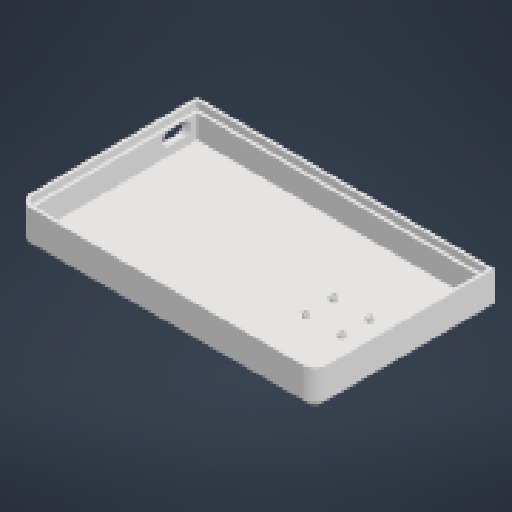
# Autodesk Inventor part: AASTRC Bottom case
Saved by Autodesk Inventor 2024 (Build 280153000, 153)
## iProperties
Created: 2023-07-16
Part Number: AASTRC Bottom case
Material: 일반
Document SubType Name: Modeling
Designer: 6gioc
Density: 1 g/cm^3
Appearance: 기본값
Mass: 597.29 g
Surface Area: 2047.87 cm^2
Volume: 597.29 cm^3
Author: 6gioc
Autodesk Inventor part; units mm, degrees
ref_plane "YZ Plane" through (0, 0, 0) normal (1, 0, 0) x (0, 1, 0)
ref_plane "XZ Plane" through (0, 0, 0) normal (0, 1, 0) x (-1, 0, 0)
ref_plane "XY Plane" through (0, 0, 0) normal (0, 0, 1) x (1, 0, 0)
sketch "스케치1" plane through (0, 0, 0) normal (0, 1, 0) x (-1, 0, 0)
  line L0 (0, 0) -> (217, 0)
  line L1 (217, 0) -> (217, -131)
  line L2 (217, -131) -> (0, -131)
  line L3 (0, -131) -> (0, 0)
  dimension "d0" = 217
  dimension "d1" = 131
  constraints: 8 end point, 2 parallel, 1 horizontal, 1 perpendicular
  measures "d0" distance of L1.end L2.end
  measures "d1" distance of L0.end L1.end
extrude "돌출1" add sketch "스케치1" along normal blind 27
sketch "스케치8" plane through (0, 27, -131) normal (0, 0, -1) x (-1, 0, 0)
  line L0 (0, -27) -> (217, -27) projected
  line L1 (217, -27) -> (217, 0) projected
  line L2 (0, 0) -> (217, 0) projected
  line L3 (0, -27) -> (0, 0) projected
  point P0 (0, -27)
extrude "돌출7" add sketch "스케치8" along normal blind 50
sketch "스케치9" plane through (0, 27, 0) normal (0, 1, 0) x (1, 0, 0)
  line L0 (0, 181) -> (-217, 181) projected
  line L1 (0, 0) -> (0, 181) projected
  line L2 (-217, 181) -> (0, 181)
  line L3 (0, 181) -> (0, 154)
  line L4 (0, 154) -> (-217, 154)
  line L5 (-217, 154) -> (-217, 181)
  point P0 (0, 10)
  dimension "d56" = 27
  constraints: 8 end point, 2 parallel, 1 horizontal, 1 perpendicular, 1 point on line
  measures "d56" distance of L2.end L3.end
extrude "돌출8" add sketch "스케치9" along normal blind 154
fillet "모깎기5" radius 10 4 edges at (-217, 181, -167.5) (0, 181, -167.5) (-217, 13.5, 0) (0, 13.5, 0)
chamfer "모따기3" distance 23 angle 45 1 edges at (-108.5, 27, -154)
shell "쉘3" thickness 10 removed faces 3 at (-141.3333, 93.6667, -154) at (-144.6667, 42.3333, -146.3333) at (-141.3333, 27, -87.3333)
sketch "스케치12" plane through (-207, 10, -171) normal (0, 0, 1) x (1, 0, 0)
  line L0 (0, 0) -> (0, 161) projected
  line L1 (197, 0) -> (0, 0) projected
  line L2 (197, 0) -> (197, 161) projected
  line L3 (197, 161) -> (0, 161) projected
  point P0 (207, -10)
extrude "돌출11" cut sketch "스케치12" against normal blind 5
sketch "스케치13" plane through (-207, 10, -10) normal (0, 1, 0) x (1, 0, 0)
  line L0 (0, 0) -> (197, 0) projected
  line L1 (197, 0) -> (197, 166) projected
  line L2 (197, 166) -> (0, 166) projected
  line L3 (0, 0) -> (0, 166) projected
  point P0 (207, -10)
extrude "돌출12" cut sketch "스케치13" against normal blind 5
chamfer "모따기4" distance 10 angle 45 1 edges at (-108.5, 5, -176)
sketch "스케치15" plane through (-207, 10, -176) normal (0, 0, 1) x (1, 0, 0)
  line L0 (73.5, 105.5) -> (123.5, 105.5)
  line L1 (123.5, 105.5) -> (123.5, 55.5)
  line L2 (123.5, 55.5) -> (73.5, 55.5)
  line L3 (73.5, 55.5) -> (73.5, 105.5)
  line L4 (197, 5) -> (0, 5) projected
  line L5 (197, 161) -> (197, 5) projected
  line L6 (0, 161) -> (197, 161) projected
  line L7 (0, 5) -> (0, 161) projected
  line L8 (197, 161) -> (197, 40) projected
  line L9 (197, 161) -> (197, 5) projected
  arc A0 (207, 161) -> (197, 171) centre (197, 161) ccw projected
  line L10 (207, -10) -> (207, 161) projected
  line L11 (207, -10) -> (-10, -10) projected
  line L12 (-10, -10) -> (-10, 161) projected
  arc A1 (0, 171) -> (-10, 161) centre (0, 161) ccw projected
  line L13 (197, 171) -> (0, 171) projected
  point P0 (98.5, 105.5)
  point P1 (73.5, 80.5)
  dimension "d85" = 50
  dimension "d86" = 50
  dimension "d87" = 197
  dimension "d88" = 156
  dimension "d89" = 98.5
  dimension "d90" = 181
  dimension "d91" = 90.5
  constraints: 8 end point, 2 midpoint, 2 parallel, 1 horizontal, 1 perpendicular
  measures "d85" distance of L1.end L2.end
  measures "d86" distance of L0.end L1.end
  measures "d87" distance of L6.start L5.start
  measures "d88" distance of L4.end L6.start
  measures "d89" distance from line of point (98.5, 105.5) L7
  measures "d90" distance between parallel lines of L11 L13
  measures "d91" distance from line of L13 point (73.5, 80.5)
extrude "돌출13" cut sketch "스케치15" against normal blind 4 contours L0 L1 L2 L3
sketch "스케치17" plane through (0, 27, -181) normal (0, 0, -1) x (-1, 0, 0)
  line L0 (133.5, 88.5) -> (133.5, 38.5) construction
  line L1 (133.5, 38.5) -> (83.5, 38.5) construction
  line L2 (83.5, 38.5) -> (83.5, 88.5) construction
  line L3 (83.5, 88.5) -> (133.5, 88.5) construction
  arc A0 (10, 154) -> (0, 144) centre (10, 144) ccw projected
  line L4 (0, -27) -> (0, 144) projected
  line L5 (0, -27) -> (217, -27) projected
  line L6 (217, -27) -> (217, 144) projected
  arc A1 (217, 144) -> (207, 154) centre (207, 144) ccw projected
  line L7 (10, 154) -> (207, 154) projected
  spline S0 degree 2 poles (123.7612, 75.7515) (121.8873, 75.1553) (119.3603, 70.6408) (119.3603, 68.4829) knots 0 0 0 1 2 2 2
  spline S1 degree 2 poles (119.3603, 68.4829) (119.3603, 65.7572) (122.2564, 61.0156) (124.5846, 60.3909) knots 0 0 0 1 2 2 2
  spline S2 degree 2 poles (124.5846, 60.3909) (123.9032, 58.0059) (120.6096, 52.9519) (118.906, 51.7594) knots 0 0 0 1 2 2 2
  spline S3 degree 2 poles (118.906, 51.7594) (117.5148, 50.7941) (115.4421, 50.7941) knots 0 0 0 1 1 1
  spline S4 degree 2 poles (115.4421, 50.7941) (113.9657, 50.7941) (112.1201, 51.5039) knots 0 0 0 1 1 1
  spline S5 degree 2 poles (112.1201, 51.5039) (110.5301, 52.2705) (109.3092, 52.2705) knots 0 0 0 1 1 1
  spline S6 degree 2 poles (109.3092, 52.2705) (108.4574, 52.2705) (105.7885, 51.22) knots 0 0 0 1 1 1
  spline S7 degree 2 poles (105.7885, 51.22) (104.1985, 50.7373) (103.517, 50.7373) knots 0 0 0 1 1 1
  spline S8 degree 2 poles (103.517, 50.7373) (101.3876, 50.7373) (99.2013, 52.5261) knots 0 0 0 1 1 1
  spline S9 degree 2 poles (99.2013, 52.5261) (95.9361, 55.4789) (92.4154, 63.8265) (92.4154, 68.3694) knots 0 0 0 1 2 2 2
  spline S10 degree 2 poles (92.4154, 68.3694) (92.4154, 73.0826) (97.8384, 80.1525) (102.0122, 80.1525) knots 0 0 0 1 2 2 2
  spline S11 degree 2 poles (102.0122, 80.1525) (104.2836, 80.1525) (106.2144, 79.1871) knots 0 0 0 1 1 1
  spline S12 degree 2 poles (106.2144, 79.1871) (107.7192, 78.2501) (109.2808, 78.2501) knots 0 0 0 1 1 1
  spline S13 degree 2 poles (109.2808, 78.2501) (110.7289, 78.2501) (111.9781, 78.7896) knots 0 0 0 1 1 1
  spline S14 degree 2 poles (111.9781, 78.7896) (115.4705, 80.1525) (116.6062, 80.1525) knots 0 0 0 1 1 1
  spline S15 degree 2 poles (116.6062, 80.1525) (119.7294, 80.1525) (122.0293, 78.1082) knots 0 0 0 1 1 1
  spline S16 degree 2 poles (122.0293, 78.1082) (123.0798, 77.0576) (123.7612, 75.7515) knots 0 0 0 1 1 1
  spline S17 degree 2 poles (108.3154, 79.8969) (108.3154, 82.7646) (110.5301, 85.5187) knots 0 0 0 1 1 1
  spline S18 degree 2 poles (110.5301, 85.5187) (112.7164, 87.9037) (115.9532, 88.4432) knots 0 0 0 1 1 1
  spline S19 degree 2 poles (115.9532, 88.4432) (115.9532, 85.0361) (113.7953, 82.4807) knots 0 0 0 1 1 1
  spline S20 degree 2 poles (113.7953, 82.4807) (111.4103, 79.8969) (108.3154, 79.8969) knots 0 0 0 1 1 1
  point P0 (0, -27)
  point P1 (108.5, 88.5)
  point P2 (133.5, 63.5)
  dimension "d1" = 131
  dimension "d96" = 50
  dimension "d97" = 50
  dimension "d98" = 181
  dimension "d99" = 217
  dimension "d100" = 108.5
  dimension "d101" = 90.5
  constraints: 2 midpoint, 2 other
  measures "d96" distance of L0.start L0.end
  measures "d97" distance of L0.end L1.end
  measures "d98" distance between parallel lines of L5 L7
  measures "d99" distance of L4.start L5.end
  measures "d100" distance from line of L6 point (108.5, 88.5)
  measures "d101" distance from line of L5 point (133.5, 63.5)
extrude "돌출14" cut sketch "스케치17" against normal blind 4 contours S0 S1 S2 S3 S4 S5 S6 S7 S8 S9 S10 S11 S12 S13 S14 S15 S16 | S17 S18 S19 S20
sketch "스케치21" plane through (0, 27, 0) normal (0, 1, 0) x (1, 0, 0)
  line L0 (-217, 10) -> (-217, 131) projected
  arc A0 (-217, 10) -> (-207, 0) centre (-207, 10) ccw projected
  line L1 (-207, 0) -> (-10, 0) projected
  arc A1 (-10, 0) -> (0, 10) centre (-10, 10) ccw projected
  line L2 (0, 10) -> (0, 131) projected
  line L3 (-212, 131) -> (-212, 10)
  arc A2 (-212, 10) -> (-207, 5) centre (-207, 10) ccw
  line L4 (-207, 5) -> (-10, 5)
  arc A3 (-10, 5) -> (-5, 10) centre (-10, 10) ccw
  line L5 (-5, 10) -> (-5, 131)
  line L6 (-207, 10) -> (-207, 166) projected
  line L7 (-207, 10) -> (-207, 131) projected
  line L8 (-217, 131) -> (-207, 131) projected
  line L9 (-217, 10) -> (-217, 131) projected
  arc A4 (-217, 10) -> (-207, 0) centre (-207, 10) ccw projected
  line L10 (-207, 0) -> (-10, 0) projected
  arc A5 (-10, 0) -> (0, 10) centre (-10, 10) ccw projected
  line L11 (0, 10) -> (0, 131) projected
  line L12 (-10, 131) -> (0, 131) projected
  line L13 (-10, 131) -> (-10, 10) projected
  line L14 (-10, 10) -> (-207, 10) projected
  point P0 (0, 0)
  dimension "d105" = 5
  constraints: 6 end point, 4 point on circle, 2 centre point, 4 other
  measures "d105" distance between parallel lines of L0 L3
extrude "돌출15" cut sketch "스케치21" against normal blind 5 contours L8 L6 L14 L13 L12 L5 A3 L4 A2 L3
sketch "스케치22" plane through (-207, 181, -154) normal (0, 0, 1) x (1, 0, 0)
  line L0 (0, 0) -> (197, 0) projected
  arc A0 (207, -10) -> (197, 0) centre (197, -10) ccw projected
  line L1 (207, -131) -> (207, -10) projected
  arc A1 (0, 0) -> (-10, -10) centre (0, -10) ccw projected
  line L2 (-10, -131) -> (-10, -10) projected
  line L3 (202, -131) -> (202, -10)
  arc A2 (202, -10) -> (197, -5) centre (197, -10) ccw
  line L4 (197, -5) -> (0, -5)
  arc A3 (0, -5) -> (-5, -10) centre (0, -10) ccw
  line L5 (-5, -10) -> (-5, -131)
  line L6 (0, -131) -> (0, -10) projected
  line L7 (0, -10) -> (197, -10) projected
  line L8 (197, -10) -> (197, -131) projected
  line L9 (207, -131) -> (197, -131) projected
  line L10 (207, -131) -> (207, -10) projected
  arc A4 (207, -10) -> (197, 0) centre (197, -10) ccw projected
  line L11 (0, 0) -> (197, 0) projected
  arc A5 (0, 0) -> (-10, -10) centre (0, -10) ccw projected
  line L12 (-10, -131) -> (-10, -10) projected
  line L13 (0, -131) -> (-10, -131) projected
  point P0 (207, -181)
  dimension "d108" = 5
  constraints: 6 end point, 4 point on circle, 2 centre point, 4 other
  measures "d108" distance between parallel lines of L0 L4
extrude "돌출16" cut sketch "스케치22" against normal blind 5 contours L5 A3 L4 A2 L3 L9 L8 L7 L6 L13
sketch "스케치23" plane through (-217, 27, -131) normal (0, 0.7071068, 0.7071068) x (1, 0, 0)
  line L0 (207, 32.5269) -> (207, 0) projected
  line L1 (10, 0) -> (10, 32.5269) projected
  line L2 (5, 0) -> (5, 32.5269)
  line L3 (212, 32.5269) -> (212, 0)
  line L4 (207, 32.5269) -> (207, 0) projected
  line L5 (207, 0) -> (212, 0) projected
  line L6 (212, 0) -> (217, 0) projected
  line L7 (217, 0) -> (217, 32.5269) projected
  line L8 (217, 32.5269) -> (212, 32.5269) projected
  line L9 (212, 32.5269) -> (207, 32.5269) projected
  line L10 (10, 0) -> (10, 32.5269) projected
  line L11 (10, 32.5269) -> (5, 32.5269) projected
  line L12 (5, 32.5269) -> (0, 32.5269) projected
  line L13 (0, 32.5269) -> (0, 0) projected
  line L14 (0, 0) -> (5, 0) projected
  line L15 (5, 0) -> (10, 0) projected
  point P0 (217, -111.7229)
  dimension "d111" = 5
  dimension "d112" = 5
  constraints: 4 end point, 2 parallel
  measures "d111" distance between parallel lines of L1 L2
  measures "d112" distance between parallel lines of L0 L3
extrude "돌출17" cut sketch "스케치23" against normal blind 5 contours L9 L3 L5 L0 | L15 L2 L11 L1
sketch "스케치24" plane through (-217, 0, -181) normal (-1, 0, 0) x (0, 0, 1)
  line L0 (29.9831, 16) -> (44.9831, 16)
  line L1 (47.4831, 13.5) -> (47.4831, 13.5)
  line L2 (44.9831, 11) -> (29.9831, 11)
  line L3 (27.4831, 13.5) -> (27.4831, 13.5)
  arc A0 (29.9831, 16) -> (27.4831, 13.5) centre (29.9831, 13.5) ccw
  arc A1 (27.4831, 13.5) -> (29.9831, 11) centre (29.9831, 13.5) ccw
  arc A2 (44.9831, 11) -> (47.4831, 13.5) centre (44.9831, 13.5) ccw
  arc A3 (47.4831, 13.5) -> (44.9831, 16) centre (44.9831, 13.5) ccw
  line L4 (171, 27) -> (171, 0) projected
  line L5 (171, 27) -> (50, 27) projected
  line L6 (27, 50) -> (50, 27) projected
  line L7 (27, 50) -> (27, 171) projected
  line L8 (0, 171) -> (27, 171) projected
  line L9 (0, 0) -> (0, 171) projected
  line L10 (171, 0) -> (0, 0) projected
  line L11 (31.4738, 8.4738) -> (8.4738, 31.4738) projected
  point P0 (181, 0)
  point P1 (47.4831, 11)
  point P2 (47.4831, 16)
  point P3 (27.4831, 11)
  point P4 (27.4831, 13.5)
  point P5 (47.4831, 13.5)
  dimension "d115" = 20
  dimension "d116" = 5
  dimension "d117" = 2.5
  dimension "d118" = 13.5
  dimension "d119" = 27
  constraints: 9 tangent, 8 end point, 8 point on circle, 6 point on line, 4 centre point, 3 equal radius, 2 parallel, 1 horizontal, 1 perpendicular
  measures "d115" distance of point (47.483, 11) point (27.483, 11)
  measures "d116" distance of point (47.483, 16) point (47.483, 11)
  measures "d117" radius of A0
  measures "d118" distance from line of L10 A2.centre
  measures "d119" distance between parallel lines of L10 L5
extrude "돌출18" cut sketch "스케치24" against normal blind 10 contours L0 A3 A2 L2 A1 A0
